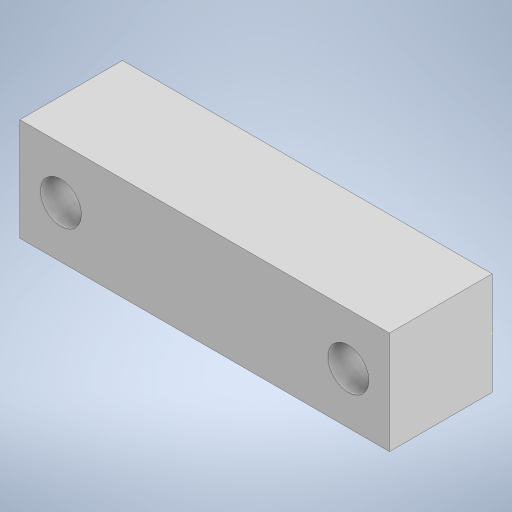
# Autodesk Inventor part: mittlere Verbindung
Saved by Autodesk Inventor 2023 (Build 270158000, 158)
## iProperties
Created: 2024-02-03
Part Number: mittlere Verbindung
Material: Generisch
Document SubType Name: Modeling
Designer: jefar
Density: 1 g/cm^3
Appearance: Vorgabe
Author: jefar
Autodesk Inventor part; units mm, degrees
ref_plane "YZ Plane" through (0, 0, 0) normal (1, 0, 0) x (0, 1, 0)
ref_plane "XZ Plane" through (0, 0, 0) normal (0, 1, 0) x (-1, 0, 0)
ref_plane "XY Plane" through (0, 0, 0) normal (0, 0, 1) x (1, 0, 0)
sketch "Skizze1" plane through (0, 0, 0) normal (0, 0, 1) x (1, 0, 0)
  line L0 (-1260, 0) -> (1260, 0) construction
  line L1 (0, -350) -> (0, 350) construction
  line L2 (-900, 250) -> (900, 250)
  line L3 (900, 250) -> (900, -250)
  line L4 (900, -250) -> (-900, -250)
  line L5 (-900, -250) -> (-900, 250)
  line L6 (-900, 250) -> (900, -250) construction
  line L7 (900, 250) -> (-900, -250) construction
  point P0 (0, 0)
  dimension "d0" = 1800
  dimension "d1" = 500
  constraints: 12 end point, 2 midpoint, 2 parallel, 1 horizontal, 1 perpendicular
  measures "d0" distance of L3.end L4.end
  measures "d1" distance of L2.end L3.end
extrude "Extrusion1" add sketch "Skizze1" along normal blind 500
sketch "Skizze2" plane through (0, 0, 0) normal (0, 0, -1) x (-1, 0, 0)
  line L0 (-900, -250) -> (-900, 250) construction
  circle A0 centre (-700, 0) radius 100
  line L1 (900, 250) -> (900, -250) projected
  circle A1 centre (700, 0) radius 100
  point P0 (0, 0)
  dimension "d5" = 200
  dimension "d7" = 200
  constraints: 2 centre point
  measures "d5" diameter of A0
  measures "d7" diameter of A1
extrude "Extrusion2" cut sketch "Skizze2" against normal through all
sketch "Skizze3" plane through (0, 0, 0) normal (0, 0, -1) x (-1, 0, 0)
  point P0 (0, 0)
sketch "Skizze4" plane through (900, -250, 0) normal (1, 0, 0) x (0, 0, -1)
  point P0 (0, 250)
